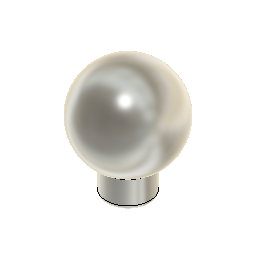
φ42シフトノブ_M12xp1.25 (Autodesk Fusion 360 design; units mm, degrees)
part number: 2025-08-30-16-58-06-209
Autodesk Fusion 360 part; units mm, degrees
sketch "スケッチ1" plane through (0, 0, 0) normal (0, 1, 0) x (1, 0, 0)
  line L0 (0, -15) -> (0, -21)
  arc A0 (0, -21) -> (10, 18.4662) centre (0, 0) ccw
  line L1 (0, -15) -> (6, -15)
  line L2 (6, -15) -> (6, 5)
  line L3 (6, 5) -> (6.75, 5)
  line L4 (6.75, 5) -> (6.75, 21)
  line L5 (10, 21) -> (10, 29)
  line L6 (8, 31) -> (6.75, 31)
  line L7 (6.75, 31) -> (6.75, 21)
  line L8 (10, 21) -> (10, 18.4662)
  arc A1 (10, 29) -> (8, 31) centre (8, 29) ccw
  dimension "d5" = 20
  dimension "d6" = 2
  constraint coincident A0.centre origin
  constraint vertical L0
  constraint perpendicular L0 L1
  constraint perpendicular L1 L2
  constraint perpendicular L4 L6
  constraint tangent L5 A1
  constraint tangent L6 A1
  measures "d5" distance of L1.end L2.end
  measures "d6" radius of A1
revolve "回転1" add sketch "スケッチ1" angle 360 about axis through (0, 0, 15) along (0, 0, 1)
thread "ねじ1" "ISO Metric profile 12.0 M12x1.25 M12x1.25 6H" major diameter 12.18 minor diameter 10.7795 pitch 1.25 angle 60 resizes the face on face at (5.9925, -0.2991, 8.3333)
chamfer "面取り1" distance 0.5 angle 45 1 edges at (-5.025, -1.949, -5)
